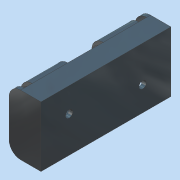
# Autodesk Inventor part: aaa_holder
Saved by Autodesk Inventor 2014 (Build 180170000, 170)
## iProperties
Created: 2013-05-29
Part Number: aaa_holder
Document SubType Name: Modeling
Designer: Administrator
Density: 1 g/cm^3
Mass: 4.5771 g
Surface Area: 65.5932 cm^2
Volume: 4.5771 cm^3
Material: Generic
Appearance: Smooth - Medium Gray
Author: Administrator
Autodesk Inventor part; units mm, degrees
ref_plane "YZ Plane" through (0, 0, 0) normal (1, 0, 0) x (0, 1, 0)
ref_plane "XZ Plane" through (0, 0, 0) normal (0, 1, 0) x (-1, 0, 0)
ref_plane "XY Plane" through (0, 0, 0) normal (0, 0, 1) x (1, 0, 0)
sketch "Sketch1" plane through (0, 0, 0) normal (0, 0, 1) x (1, 0, 0)
  line L0 (13.0048, 24.5872) -> (13.0048, 0)
  line L1 (13.0048, 0) -> (4.6736, 0)
  line L2 (13.0048, 24.5872) -> (4.6736, 24.5872)
  line L3 (0, 19.9136) -> (0, 4.6736)
  arc A0 (4.6736, 24.5872) -> (0, 19.9136) centre (4.6736, 19.9136) ccw
  arc A1 (0, 4.6736) -> (4.6736, 0) centre (4.6736, 4.6736) ccw
  point P0 (0, 0)
  dimension "d0" = 13.0048
  dimension "d1" = 24.5872
  dimension "d2" = 15.24
  constraints: 8 end point, 4 point on circle, 4 tangent, 2 centre point, 2 horizontal, 2 point on line, 1 equal radius, 1 vertical
  measures "d0" distance between parallel lines of L0 L3
  measures "d1" distance of L0.start L0.end
  measures "d2" distance of L3.start L3.end
extrude "Extrusion1" add sketch "Sketch1" along normal blind 52.9844
sketch "Sketch2" plane through (4.6736, 0, 0) normal (0, -1, 0) x (1, 0, 0)
  line L0 (0, 0) -> (0, 52.9844) projected
  line L1 (0, 1.5875) -> (-4.6736, 1.5875)
  line L2 (-4.6736, 1.5875) -> (-4.6736, 4.7625)
  line L3 (-4.6736, 4.7625) -> (0, 4.7625)
  line L4 (0, 4.7625) -> (0, 1.5875)
  line L5 (-4.6736, 19.249) -> (0, 19.249)
  line L6 (0, 19.249) -> (0, 33.7354)
  line L7 (0, 33.7354) -> (-4.6736, 33.7354)
  line L8 (-4.6736, 33.7354) -> (-4.6736, 19.249)
  line L9 (-4.6736, 48.2219) -> (0, 48.2219)
  line L10 (0, 48.2219) -> (0, 51.3969)
  line L11 (0, 51.3969) -> (-4.6736, 51.3969)
  line L12 (-4.6736, 51.3969) -> (-4.6736, 48.2219)
  line L13 (-4.6736, 0) -> (0, 0) projected
  line L14 (-4.6736, 52.9844) -> (0, 52.9844) projected
  dimension "d5" = 1.5875
  dimension "d6" = 1.5875
  dimension "d7" = 3.175
  dimension "d8" = 3.175
  dimension "d9" = 14.4865
  dimension "d10" = 14.4865
  dimension "d11" = 14.4865
  constraints: 24 end point, 3 point on line
  measures "d5" distance between parallel lines of L13 L1
  measures "d6" distance between parallel lines of L14 L11
  measures "d7" distance between parallel lines of L3 L1
  measures "d8" distance between parallel lines of L11 L9
  measures "d9" distance between parallel lines of L5 L3
  measures "d10" distance between parallel lines of L9 L7
  measures "d11" distance between parallel lines of L7 L5
extrude "Extrusion2" cut sketch "Sketch2" against normal through all
sketch "Sketch6" plane through (0, 0, 0) normal (0, 0, -1) x (-1, 0, 0)
  line L0 (-13.0048, 24.5872) -> (-13.0048, 0) projected
  line L1 (-13.0048, 0) -> (-4.6736, 0) projected
  arc A0 (-4.6736, 0) -> (0, 4.6736) centre (-4.6736, 4.6736) ccw projected
  line L2 (0, 4.6736) -> (0, 19.9136) projected
  arc A1 (0, 19.9136) -> (-4.6736, 24.5872) centre (-4.6736, 19.9136) ccw projected
  line L3 (-4.6736, 24.5872) -> (-13.0048, 24.5872) projected
  line L4 (-1.5875, 19.9136) -> (-1.5875, 4.6736)
  arc A2 (-4.6736, 1.5875) -> (-1.5875, 4.6736) centre (-4.6736, 4.6736) ccw
  line L5 (-4.6736, 1.5875) -> (-11.4173, 1.5875)
  line L6 (-11.4173, 1.5875) -> (-11.4173, 22.9997)
  line L7 (-11.4173, 22.9997) -> (-4.6736, 22.9997)
  arc A3 (-1.5875, 19.9136) -> (-4.6736, 22.9997) centre (-4.6736, 19.9136) ccw
  point P0 (0, 0)
  dimension "d14" = 1.5875
  constraints: 8 end point, 4 point on circle, 2 centre point, 5 other
  measures "d14" distance between parallel lines of L0 L6
extrude "Extrusion3" cut sketch "Sketch6" against normal up to surface (49.8094 mm away) from surface at -1.5875 contours L4 A2 L5 L6 L7 A3
sketch "Sketch7" plane through (0, 0, 0) normal (0, 0, -1) x (-1, 0, 0)
  line L0 (-13.0048, 24.5872) -> (-13.0048, 0) projected
  line L1 (-13.0048, 0) -> (-4.6736, 0) projected
  arc A0 (-4.6736, 0) -> (0, 4.6736) centre (-4.6736, 4.6736) ccw projected
  line L2 (0, 4.6736) -> (0, 19.9136) projected
  arc A1 (0, 19.9136) -> (-4.6736, 24.5872) centre (-4.6736, 19.9136) ccw projected
  line L3 (-4.6736, 24.5872) -> (-13.0048, 24.5872) projected
  line L4 (-1.5875, 23.4234) -> (-1.5875, 1.1638)
  arc A2 (-1.5875, 19.9136) -> (-4.6736, 22.9997) centre (-4.6736, 19.9136) ccw
  line L5 (-1.5875, 19.9136) -> (-1.5875, 4.6736)
  arc A3 (-4.6736, 1.5875) -> (-1.5875, 4.6736) centre (-4.6736, 4.6736) ccw
  line L6 (-4.6736, 1.5875) -> (-11.4173, 1.5875)
  line L7 (-11.4173, 1.5875) -> (-11.4173, 22.9997)
  line L8 (-11.4173, 22.9997) -> (-4.6736, 22.9997)
  arc A4 (0, 19.9136) -> (-4.6736, 22.9997) centre (-4.6736, 17.9178) ccw
  arc A5 (-4.6736, 1.5875) -> (0, 4.6736) centre (-4.6736, 6.6694) ccw
  point P0 (0, 0)
  dimension "d17" = 1.5875
  dimension "d20" = 1.5875
  constraints: 10 end point, 10 point on circle, 4 centre point, 2 tangent, 5 other
  measures "d17" distance between parallel lines of L2 L4
  measures "d20" radial gap between concentric circles of A1 A2
extrude "Extrusion4" cut sketch "Sketch7" against normal up to surface (43.4594 mm away) from surface at -4.7625 contours L2 A5 L4 A4 | L4 A2 A4 | A5 A3 L4
sketch "Sketch8" plane through (11.4173, 1.5875, 1.5875) normal (-1, 0, 0) x (0, 0, 1)
  line L0 (0, 0) -> (0, 21.4122) projected
  line L1 (0, 0) -> (49.8094, 0) projected
  line L2 (49.8094, 21.4122) -> (49.8094, 0) projected
  line L3 (0, 21.4122) -> (49.8094, 21.4122) projected
  line L4 (0, 10.3092) -> (21.59, 10.3092)
  line L5 (21.59, 10.3092) -> (21.59, 11.103)
  line L6 (21.59, 11.103) -> (0, 11.103)
  line L7 (0, 11.103) -> (0, 10.3092)
  line L8 (49.8094, 10.3092) -> (28.2194, 10.3092)
  line L9 (28.2194, 10.3092) -> (28.2194, 11.103)
  line L10 (28.2194, 11.103) -> (49.8094, 11.103)
  line L11 (49.8094, 11.103) -> (49.8094, 10.3092)
  point P0 (-1.5875, -1.5875)
  dimension "d23" = 0.7937
  dimension "d24" = 0.7937
  dimension "d25" = 10.3092
  dimension "d26" = 10.3092
  dimension "d27" = 10.3092
  dimension "d28" = 21.59
  dimension "d29" = 21.59
  constraints: 16 end point, 2 point on line
  measures "d23" distance between parallel lines of L10 L8
  measures "d24" distance between parallel lines of L6 L4
  measures "d25" distance between parallel lines of L1 L4
  measures "d26" distance between parallel lines of L3 L6
  measures "d27" distance between parallel lines of L1 L8
  measures "d28" distance from line of L0 L4.end
  measures "d29" distance from line of L2 L8.end
extrude "Extrusion5" add sketch "Sketch8" along normal blind 5.08 contours L0 L6 L5 L4 | L8 L9 L10 L2
sketch "Sketch10" plane through (11.4173, 11.8967, 1.5875) normal (0, -1, 0) x (1, 0, 0)
  line L0 (-5.08, 21.59) -> (-5.08, 0) projected
  line L1 (-11.4173, 0) -> (-5.08, 7.62)
  line L2 (-5.08, 7.62) -> (-5.08, 0)
  line L3 (-11.4173, 0) -> (-5.08, 0)
  point P0 (-11.4173, -1.5875)
  dimension "d32" = 7.62
  constraints: 6 end point, 1 point on line
  measures "d32" distance of L1.end L0.end
extrude "Extrusion6" add sketch "Sketch10" against normal up to surface (0.7938 mm away) from surface at 0
sketch "Sketch11" plane through (11.4173, 11.8967, 29.8069) normal (0, -1, 0) x (1, 0, 0)
  line L0 (-5.08, 21.59) -> (-5.08, 0) projected
  line L1 (-11.4173, 21.59) -> (-5.08, 13.97)
  line L2 (-5.08, 13.97) -> (-5.08, 21.59)
  line L3 (-5.08, 21.59) -> (-11.4173, 21.59)
  line L4 (-6.7437, 21.59) -> (-11.4173, 21.59) projected
  line L5 (-11.4173, 21.59) -> (-11.4173, 23.1775) projected
  point P0 (-11.4173, -29.8069)
  dimension "d35" = 7.62
  constraints: 6 end point, 3 point on line
  measures "d35" distance of L1.end L0.start
extrude "Extrusion7" add sketch "Sketch11" against normal up to surface (0.7937 mm away) from surface at 0
sketch "Sketch12" plane through (13.0048, 0, 0) normal (1, 0, 0) x (0, 0, -1)
  line L0 (0, 0) -> (-52.9844, 0) projected
  line L1 (0, 24.5872) -> (0, 0) projected
  circle A0 centre (-11.5062, 9.9441) radius 1.4986
  circle A1 centre (-41.4782, 14.6431) radius 1.4986
  dimension "d38" = 2.9972
  dimension "d39" = 29.972
  dimension "d40" = 4.699
  dimension "d41" = 52.9844
  dimension "d42" = 24.5872
  dimension "d43" = 9.9441
  dimension "d44" = 11.5062
  constraints: 2 centre point, 1 equal radius
  measures "d38" diameter of A0
  measures "d39" horizontal distance of A1.centre A0.centre
  measures "d40" vertical distance of A0.centre A1.centre
  measures "d41" distance of L0.start L0.end
  measures "d42" distance of L1.start L0.start
  measures "d43" distance from line of L0 A0.centre
  measures "d44" distance from line of L1 A0.centre
extrude "Extrusion8" cut sketch "Sketch12" against normal up to surface (1.5875 mm away) from surface at 0
equation "\"d9\" = d11"
equation "\"d10\" = d11"
equation "\"d24\" = d23"
equation "\"d25\" = d26"
equation "\"d27\" = d25"
equation "\"d43\" = -0.5 * d40 + 0.5 * d42"
equation "\"d44\" = -0.5 * d39 + 0.5 * d41"
body "Solid1"
